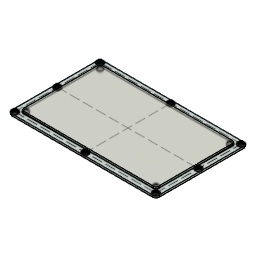
Display Mount XL - Blank (Autodesk Fusion 360 design; units mm, degrees)
Autodesk Fusion 360 part; units mm, degrees
sketch "Sketch1" plane through (0, 0, 0) normal (0, 0, 1) x (1, 0, 0)
  line L0 (-116.1, 70.1) -> (116.1, 70.1) construction
  line L1 (116.1, 70.1) -> (116.1, -70.1) construction
  line L2 (116.1, -70.1) -> (-116.1, -70.1) construction
  line L3 (-116.1, -70.1) -> (-116.1, 70.1) construction
  circle A0 centre (-116.1, 70.1) radius 1.9
  circle A1 centre (-116.1, 0) radius 1.9
  circle A2 centre (-116.1, -70.1) radius 1.9
  circle A3 centre (0, 70.1) radius 1.9
  circle A4 centre (0, -70.1) radius 1.9
  circle A5 centre (116.1, -70.1) radius 1.9
  circle A6 centre (116.1, 0) radius 1.9
  circle A7 centre (116.1, 70.1) radius 1.9
  circle A8 centre (-116.1, 70.1) radius 5.15
  circle A9 centre (-116.1, 0) radius 5.15
  circle A10 centre (-116.1, -70.1) radius 5.15
  circle A11 centre (0, -70.1) radius 5.15
  circle A12 centre (0, 70.1) radius 5.15
  circle A13 centre (116.1, 70.1) radius 5.15
  circle A14 centre (116.1, 0) radius 5.15
  circle A15 centre (116.1, -70.1) radius 5.15
  line L4 (-121.25, 70.1) -> (-121.25, -70.1)
  line L5 (-116.1, -75.25) -> (116.1, -75.25)
  line L6 (121.25, -70.1) -> (121.25, 70.1)
  line L7 (116.1, 75.25) -> (-116.1, 75.25)
  point P0 (0, 70.1)
  point P1 (-116.1, 0)
  dimension "d1" = 232.2
  dimension "d2" = 140.2
  dimension "d3" = 3.8
  dimension "d4" = 3.8
  dimension "d5" = 3.8
  dimension "d6" = 3.8
  dimension "d7" = 3.8
  dimension "d8" = 3.8
  dimension "d9" = 3.8
  dimension "d10" = 3.8
  dimension "d11" = 10.3
  dimension "d12" = 10.3
  dimension "d13" = 10.3
  dimension "d15" = 10.3
  dimension "d16" = 10.3
  dimension "d17" = 10.3
  dimension "d18" = 10.3
  dimension "d19" = 10.3
  constraint horizontal L0
  constraint vertical L1
  constraint horizontal L2
  constraint vertical L3
  constraint midpoint L0 P0
  constraint midpoint L3 P1
  constraint vertical origin A3.centre
  constraint horizontal origin P1
  constraint coincident L0.start L3.end
  constraint coincident P1 A1.centre
  constraint coincident L2.end L3.start
  constraint coincident P0 A3.centre
  constraint midpoint L2 A4.centre
  constraint coincident L1.end L2.start
  constraint midpoint L1 A6.centre
  constraint coincident L0.end L1.start
  constraint concentric A0 A8
  constraint concentric A1 A9
  constraint concentric A2 A10
  constraint concentric A4 A11
  constraint concentric A7 A13
  constraint concentric A6 A14
  constraint concentric A5 A15
  constraint coincident A8 L4.start
  constraint coincident A10 L4.end
  constraint tangent A10 L4
  constraint parallel L3 L4
  constraint coincident A10 L5.start
  constraint coincident A15 L5.end
  constraint tangent A15 L5
  constraint perpendicular L4 L5
  constraint coincident A15 L6.start
  constraint coincident A13 L6.end
  constraint tangent A13 L6
  constraint perpendicular L5 L6
  constraint coincident A13 L7.start
  constraint coincident A8 L7.end
  constraint tangent A8 L7
  constraint perpendicular L6 L7
  measures "d1" distance of L0.start L0.end
  measures "d2" distance of L0.start L2.end
  measures "d3" diameter of A0
  measures "d4" diameter of A1
  measures "d5" diameter of A2
  measures "d6" diameter of A3
  measures "d7" diameter of A4
  measures "d8" diameter of A7
  measures "d9" diameter of A6
  measures "d10" diameter of A5
  measures "d11" diameter of A8
  measures "d12" diameter of A9
  measures "d13" diameter of A10
  measures "d15" diameter of A12
  measures "d16" diameter of A13
  measures "d17" diameter of A14
  measures "d18" diameter of A15
  measures "d19" diameter of A11
extrude "Extrude1" add sketch "Sketch1" along normal blind 3 contours A8 | A9 | A11 | A14 | A12 | A8 A10 A13 A15 L4 L5 L6 L7 | A13 | A10 | A15
sketch "Sketch2" plane through (0, 0, 3) normal (0, 0, 1) x (-1, 0, 0)
  circle A0 centre (-116.1, 0) radius 1.9
  circle A1 centre (116.1, -70.1) radius 1.9
  circle A2 centre (-116.1, -70.1) radius 1.9
  circle A3 centre (0, -70.1) radius 1.9
  circle A4 centre (116.1, 0) radius 1.9
  circle A5 centre (0, 70.1) radius 1.9
  circle A6 centre (-116.1, 70.1) radius 1.9
  circle A7 centre (116.1, 70.1) radius 1.9
  line L0 (-116.1, -75.25) -> (116.1, -75.25)
  arc A8 (116.1, -75.25) -> (121.25, -70.1) centre (116.1, -70.1) ccw
  line L1 (121.25, -70.1) -> (121.25, 70.1)
  arc A9 (121.25, 70.1) -> (116.1, 75.25) centre (116.1, 70.1) ccw
  line L2 (116.1, 75.25) -> (-116.1, 75.25)
  arc A10 (-116.1, 75.25) -> (-121.25, 70.1) centre (-116.1, 70.1) ccw
  line L3 (-121.25, 70.1) -> (-121.25, -70.1)
  arc A11 (-121.25, -70.1) -> (-116.1, -75.25) centre (-116.1, -70.1) ccw
  circle A12 centre (116.1, -70.1) radius 5.15
  circle A13 centre (116.1, 0) radius 5.15
  circle A14 centre (116.1, 70.1) radius 5.15
  circle A15 centre (0, -70.1) radius 5.15
  circle A16 centre (-116.1, -70.1) radius 5.15
  circle A17 centre (-116.1, 0) radius 5.15
  circle A18 centre (-116.1, 70.1) radius 5.15
  circle A19 centre (0, 70.1) radius 5.15
  line L4 (116.1, 0) -> (-116.1, 0) construction
  line L5 (0, -70.1) -> (0, 70.1) construction
  circle A20 centre (107.1, -61.1) radius 4
  circle A21 centre (107.1, 61.1) radius 4
  circle A22 centre (-107.1, -61.1) radius 4
  circle A23 centre (-107.1, 61.1) radius 4
  line L6 (116.1, -70.1) -> (116.1, 70.1) construction
  line L7 (116.1, 70.1) -> (-116.1, 70.1) construction
  line L8 (-116.1, 70.1) -> (-116.1, -70.1) construction
  line L9 (-116.1, -70.1) -> (116.1, -70.1) construction
  line L10 (107.1, -65.1) -> (-107.1, -65.1)
  line L11 (-111.1, -61.1) -> (-111.1, 61.1)
  line L12 (-107.1, 65.1) -> (107.1, 65.1)
  line L13 (111.1, -61.1) -> (111.1, 61.1)
  dimension "d22" = 10.3
  dimension "d23" = 10.3
  dimension "d24" = 10.3
  dimension "d25" = 10.3
  dimension "d26" = 10.3
  dimension "d27" = 10.3
  dimension "d28" = 10.3
  dimension "d29" = 10.3
  dimension "d30" = 8
  dimension "d31" = 8
  dimension "d32" = 8
  dimension "d33" = 8
  dimension "d36" = 5
  dimension "d37" = 5
  constraint concentric A1 A12
  constraint concentric A4 A13
  constraint concentric A7 A14
  constraint concentric A3 A15
  constraint concentric A2 A16
  constraint concentric A0 A17
  constraint concentric A6 A18
  constraint concentric A5 A19
  constraint coincident A4.centre A13.centre
  constraint coincident A0.centre A17.centre
  constraint coincident A3.centre A15.centre
  constraint coincident A5.centre A19.centre
  constraint coincident A1.centre A8.centre
  constraint coincident A7.centre A9.centre
  constraint coincident A6.centre A10.centre
  constraint coincident A2.centre A11.centre
  constraint vertical A20.centre A21.centre
  constraint horizontal A20.centre A22.centre
  constraint vertical A22.centre A23.centre
  constraint horizontal A21.centre A23.centre
  constraint symmetric L4 A20.centre A21.centre
  constraint symmetric L5 A20.centre A22.centre
  constraint coincident A20 L10.start
  constraint coincident A22 L10.end
  constraint tangent A22 L10
  constraint tangent A20 L10
  constraint coincident A22 L11.start
  constraint coincident A23 L11.end
  constraint perpendicular L4 L11
  constraint tangent A22 L11
  constraint coincident A23 L12.start
  constraint coincident A21 L12.end
  constraint tangent A21 L12
  constraint tangent A23 L12
  constraint coincident A20 L13.start
  constraint coincident A21 L13.end
  constraint tangent A20 L13
  constraint tangent A21 L13
  measures "d22" diameter of A12
  measures "d23" diameter of A13
  measures "d24" diameter of A14
  measures "d25" diameter of A15
  measures "d26" diameter of A16
  measures "d27" diameter of A17
  measures "d28" diameter of A18
  measures "d29" diameter of A19
  measures "d30" diameter of A20
  measures "d31" diameter of A21
  measures "d32" diameter of A22
  measures "d33" diameter of A23
  measures "d36" distance of L8 L11
  measures "d37" distance of L7 L12
extrude "Extrude4" add sketch "Sketch2" along normal blind 3 contours A13 A15 A17 A19 A20 A21 A22 A23 L10 L11 L12 L13 | A22 | A20 | A23 | A21
equation "d4 = d3"
equation "d5 = d3"
equation "d6 = d3"
equation "d7 = d3"
equation "d8 = d3"
equation "d9 = d3"
equation "d10 = d3"
equation "d12 = d11"
equation "d13 = d11"
equation "d15 = d11"
equation "d16 = d11"
equation "d17 = d11"
equation "d18 = d11"
equation "d19 = d11"
equation "d22 = d11"
equation "d23 = d11"
equation "d24 = d11"
equation "d25 = d11"
equation "d26 = d11"
equation "d27 = d11"
equation "d28 = d11"
equation "d29 = d11"
equation "d31 = d30"
equation "d32 = d30"
equation "d33 = d30"
equation "d37 = d36"
